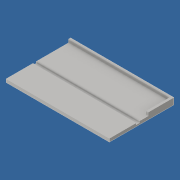
# Autodesk Inventor part: Fixture Base
Saved by Autodesk Inventor 2016 (Build 200138000, 138)
## iProperties
Created: 2016-04-07
Part Number: Fixture Base
Material: Generic
Document SubType Name: Modeling
Designer: Sam Clay
Density: 1 g/cm^3
Appearance: Default
Author: Sam Clay
Autodesk Inventor part; units mm, degrees
ref_plane "YZ Plane" through (0, 0, 0) normal (1, 0, 0) x (0, 1, 0)
ref_plane "XZ Plane" through (0, 0, 0) normal (0, 1, 0) x (-1, 0, 0)
ref_plane "XY Plane" through (0, 0, 0) normal (0, 0, 1) x (1, 0, 0)
sketch "Sketch1" plane through (0, 0, 0) normal (0, 1, 0) x (-1, 0, 0)
  line L0 (0, 0) -> (609.6, 0)
  line L1 (609.6, 0) -> (609.6, 381)
  line L2 (609.6, 381) -> (0, 381)
  line L3 (0, 381) -> (0, 0)
  dimension "d0" = 609.6
  dimension "d1" = 381
  constraints: 8 end point, 2 parallel, 1 horizontal, 1 perpendicular
  measures "d0" distance of L2.end L1.end
  measures "d1" distance of L1.end L0.end
extrude "Extrusion1" add sketch "Sketch1" along normal blind 19.05
sketch "Sketch2" plane through (0, 19.05, 0) normal (0, 1, 0) x (1, 0, 0)
  line L0 (0, 0) -> (-609.6, 0) projected
  line L1 (-609.6, 0) -> (-609.6, -381) projected
  line L2 (0, 0) -> (-609.6, 0)
  line L3 (-609.6, 0) -> (-609.6, -12.7)
  line L4 (-609.6, -12.7) -> (0, -12.7)
  line L5 (0, -12.7) -> (0, 0)
  line L6 (0, 0) -> (-12.7, 0)
  line L7 (-12.7, 0) -> (-12.7, -152.4)
  line L8 (-12.7, -152.4) -> (0, -152.4)
  line L9 (0, -152.4) -> (0, 0)
  dimension "d4" = 12.7
  dimension "d5" = 12.7
  dimension "d6" = 152.4
  constraints: 16 end point, 4 parallel, 2 horizontal, 2 perpendicular, 1 point on line
  measures "d4" distance of L3.end L2.end
  measures "d5" distance of L8.end L7.end
  measures "d6" distance of L7.end L6.end
extrude "Extrusion2" add sketch "Sketch2" along normal blind 19.05
sketch "Sketch3" plane through (0, 19.05, 0) normal (0, 1, 0) x (1, 0, 0)
  line L0 (0, -152.4) -> (0, 0) projected
  line L1 (-609.6, -12.7) -> (-609.6, -381) projected
  line L2 (0, -222.25) -> (-609.6, -222.25)
  line L3 (-609.6, -222.25) -> (-609.6, -203.2)
  line L4 (-609.6, -203.2) -> (0, -203.2)
  line L5 (0, -203.2) -> (0, -222.25)
  line L6 (0, 0) -> (-609.6, 0) projected
  dimension "d34" = 19.05
  dimension "d66" = 203.2
  constraints: 8 end point, 2 parallel, 2 point on line, 1 horizontal, 1 perpendicular
  measures "d34" distance of L2.end L3.end
  measures "d66" distance between parallel lines of L6 L4
extrude "Extrusion3" cut sketch "Sketch3" against normal blind 9.525
sketch "Sketch4" plane through (0, 19.05, 0) normal (0, 1, 0) x (1, 0, 0)
  line L0 (-609.6, -222.25) -> (-609.6, -381) projected
  line L1 (0, -374.65) -> (-609.6, -374.65)
  line L2 (-609.6, -374.65) -> (-609.6, -501.65)
  line L3 (-609.6, -501.65) -> (0, -501.65)
  line L4 (0, -501.65) -> (0, -374.65)
  point P0 (0, 0)
  dimension "d37" = 127
  dimension "d44" = 374.65
  constraints: 8 end point, 2 parallel, 1 horizontal, 1 perpendicular, 1 point on line
  measures "d37" distance of L2.end L1.end
  measures "d44" distance of point (0, 0) L1.start
extrude "Extrusion4" add sketch "Sketch4" along normal blind 12.7 separate body
body "Solid1"
body "Solid5"
